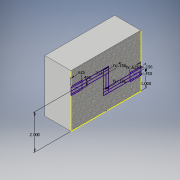
# Autodesk Inventor part: Valveblock
Saved by Autodesk Inventor 2018 (Build 220112000, 112)
## iProperties
Created: 2020-03-28
Part Number: Valveblock
Material: Generic
Document SubType Name: Modeling
Designer: emile
Density: 1 g/cm^3
Appearance: Default
Author: emile
Autodesk Inventor part; units mm, degrees
ref_plane "YZ Plane" through (0, 0, 0) normal (1, 0, 0) x (0, 1, 0)
ref_plane "XZ Plane" through (0, 0, 0) normal (0, 1, 0) x (-1, 0, 0)
ref_plane "XY Plane" through (0, 0, 0) normal (0, 0, 1) x (1, 0, 0)
sketch "Sketch1" plane through (0, 0, 0) normal (0, 1, 0) x (-1, 0, 0)
  line L0 (-38.1, 50.8) -> (38.1, 50.8)
  line L1 (38.1, 50.8) -> (38.1, -50.8)
  line L2 (38.1, -50.8) -> (-38.1, -50.8)
  line L3 (-38.1, -50.8) -> (-38.1, 50.8)
  line L4 (-38.1, 50.8) -> (38.1, -50.8) construction
  line L5 (38.1, 50.8) -> (-38.1, -50.8) construction
  point P0 (0, 0)
  dimension "d0" = 76.2
  dimension "d1" = 101.6
  constraints: 12 end point, 2 midpoint, 2 parallel, 1 horizontal, 1 perpendicular
  measures "d0" distance of L1.end L2.end
  measures "d1" distance of L2.end L0.start
extrude "Extrusion1" add sketch "Sketch1" along normal blind 76.2
sketch "Sketch2" plane through (0, 0, 0) normal (1, 0, 0) x (0, 1, 0)
  line L0 (0, 50.8) -> (76.2, 50.8) projected
  line L1 (46.8312, 50.8) -> (46.8313, -3.9688)
  line L2 (46.8313, -3.9688) -> (21.4312, -3.9688)
  line L3 (21.4312, -3.9688) -> (21.4313, -50.8)
  line L4 (0, -50.8) -> (76.2, -50.8) projected
  line L5 (29.3688, -50.8) -> (29.3687, 3.9688)
  line L6 (29.3687, 3.9688) -> (54.7688, 3.9688)
  line L7 (54.7688, 3.9688) -> (54.7688, 50.8)
  line L8 (0, 50.8) -> (0, -50.8) projected
  line L9 (21.4312, -3.9688) -> (29.3687, -3.9688)
  line L10 (21.4312, -3.9688) -> (21.4312, 3.9688)
  line L11 (54.7688, 3.9688) -> (46.8313, 3.9688)
  line L12 (54.7688, 3.9688) -> (54.7688, -3.9688)
  line L13 (25.4, 3.9688) -> (25.4, -50.8)
  line L14 (29.3687, 0) -> (46.8313, 0)
  line L15 (50.8, -3.9687) -> (50.8, 50.8)
  line L16 (54.7688, 50.8) -> (46.8312, 50.8)
  line L17 (21.4313, -50.8) -> (29.3688, -50.8)
  line L18 (45.085, 34.925) -> (45.085, 50.8)
  line L19 (45.085, 50.8) -> (56.515, 50.8)
  line L20 (56.515, 50.8) -> (56.515, 34.925)
  line L21 (56.515, 34.925) -> (45.085, 34.925)
  line L22 (45.085, 34.925) -> (56.515, 50.8) construction
  line L23 (45.085, 50.8) -> (56.515, 34.925) construction
  line L24 (19.685, -34.925) -> (19.685, -50.8)
  line L25 (19.685, -50.8) -> (31.115, -50.8)
  line L26 (31.115, -50.8) -> (31.115, -34.925)
  line L27 (31.115, -34.925) -> (19.685, -34.925)
  line L28 (19.685, -34.925) -> (31.115, -50.8) construction
  line L29 (19.685, -50.8) -> (31.115, -34.925) construction
  line L30 (50.8, 50.8) -> (50.8, 34.925)
  line L31 (25.4, -34.925) -> (25.4, -50.8)
  line L32 (29.3687, 3.9688) -> (21.4312, 3.9688)
  line L33 (46.8313, -3.9688) -> (54.7688, -3.9688)
  point P0 (0, 0)
  point P1 (21.4312, 0)
  point P2 (0, 0)
  point P3 (50.8, 42.8625)
  point P4 (25.4, -42.8625)
  dimension "d4" = 7.9375
  dimension "d7" = 3.9688
  dimension "d8" = 3.9688
  dimension "d9" = 3.9688
  dimension "d10" = 11.43
  dimension "d11" = 11.43
  dimension "d12" = 15.875
  dimension "d13" = 15.875
  dimension "d42" = 50.8
  dimension "d43" = 25.4
  constraints: 62 end point, 18 point on line, 13 perpendicular, 8 midpoint, 7 parallel, 3 collinear, 1 horizontal, 1 horizontal alignment, 1 vertical, 2 other
  measures "d4" distance between parallel lines of L6 L2
  measures "d7" distance between parallel lines of L3 L13
  measures "d8" distance between parallel lines of L2 L14
  measures "d9" distance between parallel lines of L1 L15
  measures "d10" distance of L20.end L18.start
  measures "d11" distance between parallel lines of L24 L26
  measures "d12" distance of L19.end L20.end
  measures "d13" distance of L25.end L26.end
  measures "d42" distance between parallel lines of L8 L15
  measures "d43" distance between parallel lines of L8 L13
equation "\"d7\" = 0.5 * d4"
equation "\"d8\" = d7"
equation "\"d9\" = d8"
equation "\"d11\" = d10"
equation "\"d13\" = d12"
body "Solid1"
